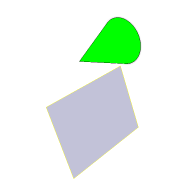
# Autodesk Inventor part: 00_lightshit_ray2
Saved by Autodesk Inventor 2019.4 (Build 234330000, 330)
## iProperties
Created: 2021-02-24
Part Number: 00_lightshit_ray2
Material: Generic
Document SubType Name: Modeling
Designer: diederichbenedict
Density: 1 g/cm^3
Appearance: Polycarbonate - Clear
Author: diederichbenedict
Autodesk Inventor part; units mm, degrees
ref_plane "YZ Plane" through (0, 0, 0) normal (1, 0, 0) x (0, 1, 0)
ref_plane "XZ Plane" through (0, 0, 0) normal (0, 1, 0) x (-1, 0, 0)
ref_plane "XY Plane" through (0, 0, 0) normal (0, 0, 1) x (1, 0, 0)
ref_plane "Work Plane1" through (14.1677, -29.8372, 1) normal (-0.9033355, -0.4289346, 0) x (0, 0, 1)
sketch "Sketch1" plane through (14.1677, -29.8372, 1) normal (-0.9033355, -0.4289346, 0) x (0, 0, 1)
  line L0 (-1, 40.53) -> (-1, 25.53) projected
  line L1 (-1, 33.03) -> (42.6224, 33.03)
  line L2 (42.6224, 33.03) -> (42.6224, 14.5833)
  line L3 (42.6224, 14.5833) -> (17.0213, 33.03)
  line L4 (-1, 25.53) -> (17.0213, 33.03)
  line L5 (-1, 25.53) -> (-1, 33.03)
  constraints: 10 end point, 2 perpendicular, 1 horizontal, 1 point on line
revolve "Revolution1" add sketch "Sketch1" angle 360 about axis through (0, 0, 0) along (0, 0, 1) contours L1 L4 L0
body "Solid1"
